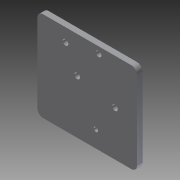
# Autodesk Inventor part: projectorMountingPlate
Saved by Autodesk Inventor 2012 (Build 160160000, 160)
## iProperties
Created: 2014-06-12
Part Number: projectorMountingPlate
Material: Default
Document SubType Name: Modeling
Designer: Byron
Density: 1 g/cm^3
Author: Byron
Autodesk Inventor part; units mm, degrees
ref_plane "YZ Plane" through (0, 0, 0) normal (1, 0, 0) x (0, 1, 0)
ref_plane "XZ Plane" through (0, 0, 0) normal (0, 1, 0) x (-1, 0, 0)
ref_plane "XY Plane" through (0, 0, 0) normal (0, 0, 1) x (1, 0, 0)
sketch "Sketch1" plane through (0, 0, 0) normal (0, 0, 1) x (1, 0, 0)
  circle A0 centre (-45.2437, 35.97) radius 1.27 projected
  circle A1 centre (-45.2437, 35.97) radius 1.27 projected
  circle A2 centre (10.6363, 0) radius 3.175 projected
  line L0 (-76.9938, -50.8) -> (-76.9938, 50.8) projected
  line L1 (76.9938, -50.8) -> (-76.9938, -50.8) projected
  line L2 (76.9938, 50.8) -> (76.9938, -50.8) projected
  line L3 (-76.9938, 50.8) -> (76.9938, 50.8) projected
  line L4 (-70.6437, 50.8) -> (29.0843, 50.8)
  line L5 (35.4343, 44.45) -> (35.4343, -44.45)
  line L6 (29.0843, -50.8) -> (-70.6437, -50.8)
  line L7 (-76.9937, -44.45) -> (-76.9938, 44.45)
  arc A3 (-70.6437, 50.8) -> (-76.9938, 44.45) centre (-70.6437, 44.45) ccw
  arc A4 (29.0843, -50.8) -> (35.4343, -44.45) centre (29.0843, -44.45) ccw
  arc A5 (35.4343, 44.45) -> (29.0843, 50.8) centre (29.0843, 44.45) ccw
  arc A6 (-76.9937, -44.45) -> (-70.6437, -50.8) centre (-70.6437, -44.45) ccw
  circle A7 centre (-7.7961, 43.4062) radius 3.175 projected
  circle A8 centre (-32.0501, 9.7076) radius 3.175 projected
  point P0 (0, 0)
  point P1 (35.4343, -50.8)
  dimension "d0" = 6.35
  constraints: 8 end point, 8 point on circle, 8 tangent, 5 point on line, 4 centre point, 3 equal radius, 2 parallel, 1 horizontal, 1 perpendicular
  measures "d0" radius of A3
extrude "Extrusion1" add sketch "Sketch1" along normal blind 6.35 contours L0 A3 L3 A5 L5 A4 L1 A6 | A7 | A8
sketch "Sketch2" plane through (0, 0, 6.35) normal (0, 0, 1) x (1, 0, 0)
  circle A0 centre (-45.2437, 35.97) radius 1.27 projected
  circle A1 centre (-7.7961, 43.4062) radius 3.175 projected
  circle A2 centre (-32.0501, 9.7076) radius 3.175 projected
  circle A3 centre (-45.2437, 35.97) radius 3.175 projected
  point P0 (0, 0)
extrude "Extrusion2" cut sketch "Sketch2" against normal through all
sketch "Sketch3" plane through (0, 0, 6.35) normal (0, 0, 1) x (1, 0, 0)
  arc A0 (-12.0087, -29.8172) -> (-8.9086, -33.4326) centre (-11.0366, -32.1205) ccw projected
  circle A1 centre (-11.0366, -32.1205) radius 2.5
  point P0 (0, 0)
  constraints: 1 centre point, 1 coincident, 1 concentric
extrude "Extrusion3" cut sketch "Sketch3" against normal through all
body "Solid1"
